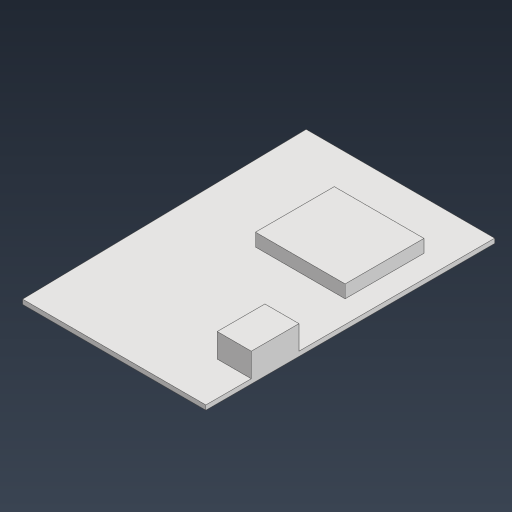
# Autodesk Inventor part: adc
Saved by Autodesk Inventor 2023 (Build 270158000, 158)
## iProperties
Created: 2025-06-15
Part Number: adc
Material: Generic
Document SubType Name: Modeling
Designer: szymo
Density: 1 g/cm^3
Appearance: Default
Author: szymo
Autodesk Inventor part; units mm, degrees
ref_plane "YZ Plane" through (0, 0, 0) normal (1, 0, 0) x (0, 1, 0)
ref_plane "XZ Plane" through (0, 0, 0) normal (0, 1, 0) x (-1, 0, 0)
ref_plane "XY Plane" through (0, 0, 0) normal (0, 0, 1) x (1, 0, 0)
sketch "Sketch1" plane through (0, 0, 0) normal (0, 1, 0) x (-1, 0, 0)
  line L0 (0, 0) -> (24.2, 0)
  line L1 (24.2, 0) -> (24.9, -38.1436)
  line L2 (24.9, -38.1436) -> (0, -38.1436)
  line L3 (0, -38.1436) -> (0, 0)
  dimension "d0" = 38.15
  dimension "d1" = 24.9
  dimension "d2" = 24.2
  constraints: 8 end point, 1 horizontal, 1 parallel, 1 vertical
  measures "d0" distance of L0.end L1.end
  measures "d1" distance of L2.end L1.end
  measures "d2" distance of L0.start L0.end
extrude "Extrusion1" add sketch "Sketch1" along normal blind 0.6
sketch "Sketch2" plane through (0, 0.6, 0) normal (0, 1, 0) x (1, 0, 0)
  line L0 (0, 38.1436) -> (-24.9, 38.1436) projected
  line L1 (-24.9, 38.1436) -> (-24.2, 0) projected
  line L2 (-24.2, 0) -> (0, 0) projected
  line L3 (0, 0) -> (0, 38.1436) projected
  line L4 (0, 6) -> (-4.5, 6)
  line L5 (-4.5, 6) -> (-4.5, 12.3)
  line L6 (-4.5, 12.3) -> (0, 12.3)
  line L7 (0, 12.3) -> (0, 6)
  point P0 (0, 12.3)
  dimension "d5" = 4.5
  dimension "d6" = 6.3
  dimension "d7" = 6
  dimension "d8" = 25.8436
  constraints: 8 end point, 2 parallel, 1 horizontal, 1 perpendicular, 1 point on line
  measures "d5" distance of L5.end L6.end
  measures "d6" distance of L4.end L5.end
  measures "d7" distance between parallel lines of L2 L4
  measures "d8" distance between parallel lines of L0 L6
extrude "Extrusion2" add sketch "Sketch2" along normal blind 3.15 contours L3 L4 L5 L6
sketch "Sketch3" plane through (0, 0.6, 0) normal (0, 1, 0) x (1, 0, 0)
  line L0 (-14.7887, 21.3392) -> (-2.9463, 21.3392)
  line L1 (-2.9463, 21.3392) -> (-2.9463, 31.7514)
  line L2 (-2.9463, 31.7514) -> (-14.7887, 31.7514)
  line L3 (-14.7887, 31.7514) -> (-14.7887, 21.3392)
  point P0 (0, 0)
  constraints: 8 end point, 2 parallel, 1 horizontal, 1 perpendicular
extrude "Extrusion3" add sketch "Sketch3" along normal blind 1.7
body "Solid1"
